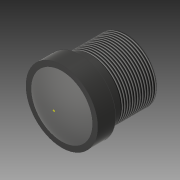
# Autodesk Inventor part: Linse 12mm Typ G
Saved by Autodesk Inventor 2019.1 (Build 231200000, 200)
## iProperties
Part Number: Linse 12mm Typ G
Material: PC/ABS-Kunststoff
Document SubType Name: Modeling
Designer: rYan
Mass: 0.587088 g
Surface Area: 8.08175 cm^2
Volume: 1.64325 cm^3
Density: 0.357273 g/cm^3
Appearance: Glatt - weiß
Author: rYan
Autodesk Inventor part; units mm, degrees
ref_plane "YZ Plane" through (0, 0, 0) normal (1, 0, 0) x (0, 1, 0)
ref_plane "XY Plane" through (0, 0, 0) normal (0, 0, 1) x (1, 0, 0)
sketch "Skizze1" plane through (0, 0, 0) normal (1, 0, 0) x (0, 1, 0)
  line L0 (0, 0) -> (-14, 0)
  line L1 (-9, 7) -> (-12.5, 7)
  line L2 (-9, 7) -> (-9, 6)
  line L3 (-9, 6) -> (0, 6)
  line L4 (0, 6) -> (0, 0)
  line L5 (-12.5, 7) -> (-12.5, 6)
  arc A0 (-12.5, 6) -> (-14, 0) centre (-1.25, 0) ccw
  dimension "d0" = 14
  dimension "d1" = 3.5
  dimension "d2" = 9
  dimension "d3" = 12
  dimension "d4" = 14
  constraints: 12 end point, 2 horizontal, 2 perpendicular, 2 point on circle, 2 point on line, 2 vertical, 1 centre point
  measures "d0" distance of L0.start L0.end
  measures "d1" distance of L1.start L1.end
  measures "d2" distance of L2.end L3.end
  measures "d3" diameter of L3 L0
  measures "d4" diameter of L1 L0
revolve "Umdrehung1" add sketch "Skizze1" angle 360 about axis through (0, 0, 0) along (0, -1, 0)
thread "Gewinde1" size "M12x0.5" class "6g" standard "ANSI Metric M Profile" length 8 offset 2
ref_plane "Arbeitsebene1" through (0, -14, 0) normal (0, 1, 0) x (-1, 0, 0)
